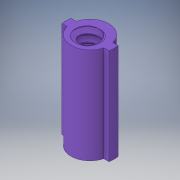
# Autodesk Inventor part: SpindleThreadLong
Saved by Autodesk Inventor 2019.1 (Build 231200000, 200)
## iProperties
Created: 2018-07-24
Part Number: SpindleThreadLong
Material: Generisch
Document SubType Name: Modeling
Designer: JochenAlt
Density: 1 g/cm^3
Appearance: Kühles Weiß
Author: JochenAlt
Autodesk Inventor part; units mm, degrees
ref_plane "YZ Plane" through (0, 0, 0) normal (1, 0, 0) x (0, 1, 0)
ref_plane "XZ Plane" through (0, 0, 0) normal (0, 1, 0) x (-1, 0, 0)
ref_plane "XY Plane" through (0, 0, 0) normal (0, 0, 1) x (1, 0, 0)
sketch "Skizze1" plane through (0, 0, 0) normal (0, 0, 1) x (1, 0, 0)
  circle A0 centre (0, 0) radius 4.5
  line L0 (0, -8.26) -> (0, 8.26) construction
  line L1 (-10.5, 0) -> (10.5, 0) construction
  arc A1 (-5.7253, -1.425) -> (5.7253, -1.425) centre (0, 0) ccw
  arc A2 (5.7253, 1.425) -> (-5.7253, 1.425) centre (0, 0) ccw
  line L2 (7.3634, 1.425) -> (5.7253, 1.425)
  line L3 (5.7253, -1.425) -> (7.3634, -1.425)
  line L4 (-5.7253, 1.425) -> (-7.3634, 1.425)
  line L5 (-7.3634, -1.425) -> (-5.7253, -1.425)
  arc A3 (-7.3634, 1.425) -> (-7.3634, -1.425) centre (0, 0) ccw
  arc A4 (7.3634, -1.425) -> (7.3634, 1.425) centre (0, 0) ccw
  dimension "d1" = 9
  dimension "d82" = 5.9
  dimension "d84" = 2.85
  dimension "d86" = 7.5
  constraints: 8 end point, 8 point on circle, 5 centre point, 3 coincident, 2 collinear, 2 concentric, 2 horizontal, 2 parallel, 1 other
  measures "d1" diameter of A0
  measures "d82" radius of A2
  measures "d84" distance of L2.start L3.end
  measures "d86" radius of A3
extrude "Extrusion1" add sketch "Skizze1" along normal blind 30
thread "Gewinde1" size "G41.91x2.309" designation "G 1 1/4" standard "GB Pipe Threads without seal" full length
sketch "Skizze9" plane through (0, 0, 30) normal (-1, 0, 0) x (0, 1, 0)
  line L0 (4.5, 0) -> (4.5, 30)
  line L1 (4.5, 30) -> (2.9931, 30)
  line L2 (2.9931, 30) -> (2.9931, 0)
  line L3 (2.9931, 0) -> (4.5, 0)
  line L4 (0, -6) -> (0, 36) projected
  line L5 (-5.9, 0) -> (-1.425, 0) projected
  line L6 (-1.425, 30) -> (-5.9, 30) construction
  constraints: 8 end point, 2 point on line
revolve "Umdrehung4" add sketch "Skizze9" angle 360 about axis through (0, 0, 30) along (0, 0, -1) separate body
sketch "Skizze8" plane through (0, 4.5, 30) normal (1, 0, 0) x (0, 0, -1)
  line L0 (-1.3072, 0.0833) -> (-1.1546, 0.0833) construction
  line L1 (0.1525, -1.4181) -> (-0.0001, -1.6877) construction
  line L2 (-2.3092, -1.6877) -> (-2.4618, -1.4181) construction
  line L3 (-1.0021, 0.0833) -> (-1.1546, 0.3529) construction
  line L4 (-1.1546, 0.3529) -> (-1.3072, 0.0833) construction
  line L5 (-2.3092, -1.6877) -> (-2.1566, -1.4181) construction
  line L6 (-1.0021, 0.0833) -> (-0.1527, -1.4181)
  line L7 (-2.4618, -1.4181) -> (-2.1566, -1.4181) construction
  arc A0 (-2.4618, -1.4181) -> (-2.3092, -1.507) centre (-2.3092, -1.3318) ccw construction
  line L8 (0.1525, -1.4181) -> (-0.1527, -1.4181) construction
  line L9 (-2.3092, -1.6877) -> (-2.3092, -1.4181) construction
  line L10 (-0.0001, -1.6877) -> (-0.0001, -1.4181) construction
  line L11 (-1.1546, 0.3529) -> (-1.1546, 0.1723) construction
  line L12 (-2.3092, -1.507) -> (-0.0001, -1.507)
  arc A1 (-2.3092, -1.507) -> (-2.1566, -1.4181) centre (-2.3092, -1.3318) ccw
  line L13 (-0.1527, -1.4181) -> (-0.0001, -1.6877) construction
  line L14 (-2.1566, -1.4181) -> (-1.3072, 0.0833)
  line L15 (-0.0001, -0.0002) -> (-0.0001, 0.0177)
  line L16 (-0.0001, 0.0177) -> (-0.0001, -0.0002)
  line L17 (-0.0001, -0.0002) -> (0.0334, -0.0002)
  arc A2 (-0.1527, -1.4181) -> (-0.0001, -1.507) centre (-0.0001, -1.3318) ccw
  arc A3 (-0.0001, -1.507) -> (0.1525, -1.4181) centre (-0.0001, -1.3318) ccw construction
  arc A4 (-1.1546, 0.1723) -> (-1.3072, 0.0833) centre (-1.1546, -0.003) ccw
  arc A5 (-1.0021, 0.0833) -> (-1.1546, 0.1723) centre (-1.1546, -0.003) ccw
  line L18 (-1.1546, 0.1723) -> (-1.1546, 0.0833) construction
  line L19 (-1.1546, 0.0833) -> (-1.0021, 0.0833) construction
  dimension "d60" = 59
  dimension "d61" = 0.2697
  dimension "d62" = 0.2697
  dimension "Skizze8_ThreadOffset" = 0
  dimension "Skizze8_MajorRadius" = 1.5069
  dimension "d65" = 2.3091
  dimension "Skizze8_MinorRadius" = 0.1724
  constraints: 40 end point, 12 point on circle, 10 parallel, 8 tangent, 6 centre point, 6 collinear, 2 midpoint, 2 point on line, 1 horizontal, 1 perpendicular, 3 other
  measures "d60" angle of L6 L14
  measures "d61" distance of L3.end L0.end
  measures "d62" distance of L1.end L10.end
  measures "Skizze8_ThreadOffset" distance between parallel lines of L15 L10
  measures "Skizze8_MajorRadius" distance from line of L12 L15.start
  measures "d65" distance from line of L1.end L9
  measures "Skizze8_MinorRadius" distance edge to line of A5 L17
coil "Spirale4" sketch "Skizze8" operation cut axis through (0, 0, 30) along (0, 0, -1) pitch 2.3114 turns 14.977149 hand right bodies 2
combine bodies "Kombinieren4" operation type add bodies to combine 1 2
equation "\"d65\" = Skizze8_Pitch"
equation "\"d13\" = 60deg"
equation "\"Skizze2_Pitch\" = 2.30909"
equation "\"d31\" = 60deg"
equation "\"Skizze4_Pitch\" = 2.30909"
equation "\"d49\" = 60deg"
equation "\"Skizze6_Pitch\" = 2.30909"
equation "\"d67\" = 60deg"
equation "\"Skizze8_Pitch\" = 2.30909"
